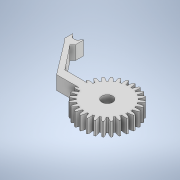
# Autodesk Inventor part: New Gear
Saved by Autodesk Inventor 2022 (Build 260153000, 153)
## iProperties
Created: 2022-02-25
Part Number: New Gear
Material: Generic
Document SubType Name: Modeling
Designer: Alexa
Density: 1 g/cm^3
Appearance: Default
Author: Alexa
Autodesk Inventor part; units mm, degrees
ref_plane "YZ Plane" through (0, 0, 0) normal (1, 0, 0) x (0, 1, 0)
ref_plane "XZ Plane" through (0, 0, 0) normal (0, 1, 0) x (-1, 0, 0)
ref_plane "XY Plane" through (0, 0, 0) normal (0, 0, 1) x (1, 0, 0)
sketch "Sketch1" plane through (0, 0, 0) normal (0, 1, 0) x (-1, 0, 0)
  circle A0 centre (0, 0) radius 8
  circle A1 centre (0, 0) radius 2
  line L0 (7.9113, 0.5933) -> (7.9113, -0.6067)
  line L1 (9.9113, -0.2567) -> (9.9113, 0.2433)
  line L2 (7.6237, -0.0067) -> (9.0479, -0.0067) construction
  arc A2 (9.9113, 0.2433) -> (7.9113, 0.5933) centre (8.1555, -3.9001) ccw construction
  arc A3 (7.9113, -0.6067) -> (9.9113, -0.2567) centre (8.1555, 3.8866) ccw construction
  arc A4 (9.9113, 0.2433) -> (7.9113, 0.5933) centre (8.1555, -3.9001) ccw construction
  arc A5 (9.9113, 0.2433) -> (7.9777, 0.5964) centre (8.1555, -3.9001) ccw
  arc A6 (7.9767, -0.6098) -> (9.9113, -0.2567) centre (8.1555, 3.8866) ccw
  line L3 (9.4, 0) -> (9.4, -0.4379)
  line L4 (9.4, 0) -> (9.4, 0.4244)
  arc A7 (5.296, -1.8919) -> (5.296, 1.8784) centre (4.6281, -0.0067) ccw
  circle A8 centre (0, 0) radius 8
  dimension "d0" = 16
  dimension "d1" = 4
  dimension "d2" = 0.25
  dimension "d3" = 0.25
  dimension "d4" = 0.6
  dimension "d7" = 1.2
  dimension "d8" = 4.5
  dimension "d10" = 2
  constraints: 18 point on circle, 10 end point, 9 centre point, 4 concentric, 3 coincident, 2 vertical, 1 horizontal, 1 parallel, 1 point on line
  measures "d0" diameter of A0
  measures "d1" diameter of A1
  measures "d2" distance from line of L1.start L2
  measures "d3" distance from line of L1.end L2
  measures "d4" distance from line of L0.start L2
  measures "d7" distance of L0.end L0.start
  measures "d8" radius of A3
  measures "d10" radius of A7
extrude "Extrusion1" add sketch "Sketch1" along normal blind 5
pattern_circular "Circular Pattern1" count 28 over 360 about axis through (0, 0, 0) along (0, 1, 0) of "Extrusion1"
sketch "Sketch2" plane through (0, 5, 0) normal (0, 1, 0) x (1, 0, 0)
  circle A0 centre (-4, 0) radius 1.5
  line L0 (0, 0) -> (-25, 0)
  line L1 (-25, 0) -> (-25, 28.759)
  line L2 (-25, 28.759) -> (0, 28.759)
  line L3 (0, 28.759) -> (0, 0)
  line L4 (0, 0) -> (-25, 0)
  line L5 (-25, 0) -> (-25, 14.3795)
  line L6 (-25, 14.3795) -> (0, 14.3795)
  line L7 (0, 14.3795) -> (0, 0)
  line L8 (-4, -1.5) -> (-25, -1.5)
  line L9 (-25, -1.5) -> (-25, 1.5)
  line L10 (-25, 1.5) -> (-4, 1.5)
  line L11 (-4, 1.5) -> (-4, -1.5)
  line L12 (-27, -1.5) -> (-23, -1.5)
  line L13 (-23, -1.5) -> (-23, 14.3795)
  line L14 (-23, 14.3795) -> (-27, 14.3795)
  line L15 (-27, 14.3795) -> (-27, -1.5)
  circle A1 centre (-25, 14.3795) radius 1
  line L16 (-27, -1.5) -> (-23, -1.5)
  line L17 (-23, -1.5) -> (-23, 12.5)
  line L18 (-23, 12.5) -> (-27, 12.5)
  line L19 (-27, 12.5) -> (-27, -1.5)
  line L20 (-27, 12.5) -> (-26, 14.3795)
  line L21 (-23, 12.5) -> (-24, 14.3795)
  arc A2 (-7.9777, -0.5964) -> (-7.9124, -1.1805) centre (0, 0) ccw projected
  line L22 (-7.9124, -1.1805) -> (-7.9777, -0.5964)
  line L23 (-25, -1.5) -> (-11, -1.5)
  line L24 (-11, -1.5) -> (-11, 1.5)
  line L25 (-11, 1.5) -> (-25, 1.5)
  line L26 (-25, 1.5) -> (-25, -1.5)
  point P0 (-23, 1.5)
  dimension "d16" = 3
  dimension "d17" = 25
  dimension "d18" = 28.759
  dimension "d19" = 4
  dimension "d20" = 2
  dimension "d21" = 14
  dimension "d22" = 14
  constraints: 54 end point, 12 parallel, 7 point on line, 6 horizontal, 6 perpendicular, 2 point on circle, 1 centre point, 1 coincident, 1 midpoint, 1 vertical alignment, 2 other
  measures "d17" distance of L1.end L2.end
  measures "d18" distance of L0.end L1.end
  measures "d19" distance of L14.end L13.end
  measures "d20" diameter of A1
  measures "d21" distance of L17.end L16.end
  measures "d22" distance of L25.end L24.end
extrude "Extrusion2" add sketch "Sketch2" against normal blind 5 contours L24 L0 L13 L10 | L8 L13 L0 L24 | L13 L0 L1 L10 | L10 L1 L18 L13 | L8 L9 L0 L13 | L1 L9 L12 L15 L18 | L18 L1 A1 L21 | L18 L20 A1 L1
sketch "Sketch3" plane through (-11, 5, 1.5) normal (1, 0, 0) x (0, 0, -1)
  line L0 (0, 0) -> (3, 0) projected
  line L1 (3, 0) -> (3, -5) projected
  line L2 (0, 0) -> (3, 0)
  line L3 (3, 0) -> (3, -5)
  line L4 (3, -5) -> (0, -5)
  line L5 (0, -5) -> (0, 0)
  point P0 (1.5, -5)
  dimension "d25" = 5
  constraints: 8 end point, 2 parallel, 1 horizontal, 1 perpendicular
  measures "d25" distance of L2.end L1.end
extrude "Extrusion3" add sketch "Sketch3" along normal blind 5
sketch "Sketch5" plane through (0, 5, 0) normal (0, 1, 0) x (1, 0, 0)
  line L0 (-27, -1.5) -> (-8.9321, -1.5) projected
  line L1 (-23, 1.5) -> (-8.8997, 1.5) projected
  line L2 (-27, -1.5) -> (-17, -1.5)
  line L3 (-17, -1.5) -> (-17, 1.5)
  line L4 (-17, 1.5) -> (-27, 1.5)
  line L5 (-27, 1.5) -> (-27, -1.5)
  line L6 (-17, 1.5) -> (-23, 12.5)
  line L7 (-27, -1.5) -> (-27, 12.5) projected
  line L8 (-23, 12.5) -> (-27, 12.5)
  line L9 (-17, 1.5) -> (-20, 1.5)
  line L10 (-20, 1.5) -> (-27, 12.5)
  line L11 (-28.8478, -8.4167) -> (-17, -8.4167)
  line L12 (-17, -8.4167) -> (-17, 15.7727)
  line L13 (-17, 15.7727) -> (-28.8478, 15.7727)
  line L14 (-28.8478, 15.7727) -> (-28.8478, -8.4167)
  point P0 (0, 0)
  dimension "d29" = 10
  dimension "d30" = 3
  constraints: 24 end point, 4 parallel, 3 perpendicular, 2 horizontal, 2 point on line
  measures "d29" distance of L4.end L3.end
  measures "d30" distance of L3.end L9.end
extrude "Extrusion4" cut sketch "Sketch5" against normal blind 9.05
sketch "Sketch7" plane through (0, 5, 0) normal (0, 1, 0) x (1, 0, 0)
  line L0 (0, 0) -> (-25, 0)
  line L1 (-25, 0) -> (-25, 28.759)
  line L2 (-25, 28.759) -> (0, 28.759)
  line L3 (0, 28.759) -> (0, 0)
  line L4 (-25, 0) -> (0, 0)
  line L5 (0, 0) -> (0, 14.3795)
  line L6 (0, 14.3795) -> (-25, 14.3795)
  line L7 (-25, 14.3795) -> (-25, 0)
  circle A0 centre (-25, 14.3795) radius 1
  line L8 (-17, -1.5) -> (-17, 1.5) projected
  circle A1 centre (-17, 0) radius 1.5
  line L9 (-25, 14.3795) -> (-26, 14.3795)
  line L10 (-26, 14.3795) -> (-26, 10.3795)
  line L11 (-26, 10.3795) -> (-25, 10.3795)
  line L12 (-25, 10.3795) -> (-25, 14.3795)
  line L13 (-25, 10.3795) -> (-24, 10.3795)
  line L14 (-24, 10.3795) -> (-24, 14.3795)
  line L15 (-24, 14.3795) -> (-25, 14.3795)
  line L16 (-25, 14.3795) -> (-25, 10.3795)
  line L17 (-26, 10.3795) -> (-17, -1.5)
  line L18 (-24, 10.3795) -> (-17, 1.5)
  dimension "d45" = 2
  dimension "d43" = 25
  dimension "d44" = 28.759
  dimension "d46" = 4
  constraints: 36 end point, 8 parallel, 4 horizontal, 4 perpendicular, 2 midpoint, 1 coincident, 1 point on line, 1 vertical alignment, 5 other
  measures "d43" distance of L1.end L2.end
  measures "d44" distance of L0.end L1.end
  measures "d46" distance of L10.end L9.end
extrude "Extrusion5" add sketch "Sketch7" against normal blind 5 contours L8 L17 L0 | L0 L17 A1 L8 | A1 L17 L1 L13 L18 | L14 L13 L1 A0 | L1 L11 L10 A0 | L17 L11 L1
sketch "Sketch8" plane through (0, 5, 0) normal (0, 1, 0) x (1, 0, 0)
  line L0 (-26, 10.3795) -> (-26, 14.3795) projected
  line L1 (-26, 14.3795) -> (-27, 14.3795)
  line L2 (-27, 14.3795) -> (-27, 11.3795)
  line L3 (-27, 11.3795) -> (-26, 11.3795)
  line L4 (-26, 11.3795) -> (-26, 14.3795)
  line L5 (-26, 10.3795) -> (-27, 11.3795)
  arc A0 (-26, 14.3795) -> (-24, 14.3795) centre (-25, 14.3795) ccw projected
  line L6 (-24, 14.3795) -> (-23, 14.3795)
  line L7 (-23, 14.3795) -> (-23, 11.3795)
  line L8 (-23, 11.3795) -> (-24, 11.3795)
  line L9 (-24, 11.3795) -> (-24, 14.3795)
  line L10 (-17, 1.5) -> (-24, 10.3795) projected
  line L11 (-24, 10.3795) -> (-23, 11.3795)
  line L12 (-24, 10.3795) -> (-24, 14.3795) projected
  line L13 (-24, 11.3795) -> (-24, 10.3795)
  point P0 (0, 0)
  dimension "d49" = 1
  dimension "d50" = 3
  dimension "d51" = 1
  dimension "d52" = 3
  constraints: 22 end point, 4 parallel, 2 horizontal, 2 perpendicular, 1 collinear
  measures "d49" distance of L3.end L2.end
  measures "d50" distance of L2.end L1.end
  measures "d51" distance of L7.end L8.end
  measures "d52" distance of L6.end L7.end
extrude "Extrusion6" add sketch "Sketch8" against normal blind 5
sketch "Sketch9" plane through (0, 5, 0) normal (0, 1, 0) x (1, 0, 0)
  arc A0 (-26, 14.3795) -> (-24, 14.3795) centre (-25, 14.3795) ccw projected
  circle A1 centre (-25, 14.3795) radius 2
  circle A2 centre (-25, 14.3795) radius 1.5
  line L0 (-27, 11.3795) -> (-26, 10.3795) projected
  line L1 (-23, 11.3795) -> (-23, 14.3795) projected
  line L2 (-27, 11.3795) -> (-23, 11.3795)
  line L3 (-23, 11.3795) -> (-23, 13.7795)
  line L4 (-23, 13.7795) -> (-27, 13.7795)
  line L5 (-27, 13.7795) -> (-27, 11.3795)
  line L6 (-27, 14.3795) -> (-26.3748, 13.7795)
  line L7 (-23, 14.3795) -> (-24, 14.3795) projected
  line L8 (-23, 14.3795) -> (-23.6252, 13.7795)
  point P0 (0, 0)
  point P1 (-25.8, 13.7795)
  point P2 (-24.2, 13.7795)
  dimension "d55" = 4
  dimension "d56" = 3
  dimension "d57" = 2.4
  constraints: 12 end point, 3 point on circle, 3 point on line, 2 centre point, 2 coincident, 2 parallel, 1 horizontal, 1 perpendicular
  measures "d55" diameter of A1
  measures "d56" diameter of A2
  measures "d57" distance of L3.end L2.end
extrude "Extrusion7" cut sketch "Sketch9" against normal through all contours L4 A2 L7 A0 | A0 L4 A2 | A0 L7 A2 L4 | L6 A1 L7 A2 | A2 L7 L8
body "Solid1"
